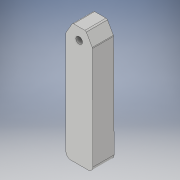
# Autodesk Inventor part: real arm
Saved by Autodesk Inventor 2019 (Build 230136000, 136)
## iProperties
Created: 2019-10-24
Part Number: real arm
Material: Generic
Document SubType Name: Modeling
Designer: robgr
Density: 1 g/cm^3
Appearance: Default
Author: robgr
Autodesk Inventor part; units mm, degrees
ref_plane "YZ Plane" through (0, 0, 0) normal (1, 0, 0) x (0, 1, 0)
ref_plane "XZ Plane" through (0, 0, 0) normal (0, 1, 0) x (-1, 0, 0)
ref_plane "XY Plane" through (0, 0, 0) normal (0, 0, 1) x (1, 0, 0)
sketch "Sketch1" plane through (0, 0, 0) normal (0, 0, 1) x (1, 0, 0)
  circle A0 centre (0, 0) radius 2
  line L0 (-8, 0) -> (-8, -65)
  line L1 (-8, -65) -> (8.3, -65)
  line L2 (8.3, -65) -> (8, 0)
  line L3 (-8, 0) -> (-4, 6.9282)
  line L4 (-4, 6.9282) -> (4, 6.9282)
  line L5 (4, 6.9282) -> (8, 0)
  dimension "d0" = 4
  dimension "d2" = 65
  dimension "d3" = 16.3
  constraints: 12 end point, 2 coincident, 1 centre point, 1 horizontal, 1 vertical, 6 other
  measures "d0" diameter of A0
  measures "d2" distance of L0.start L0.end
  measures "d3" distance of L0.end L1.end
extrude "Extrusion1" add sketch "Sketch1" along normal blind 12.75
fillet "Fillet1" radius 1 4 edges at (-4, 6.9282, 6.375) (4, 6.9282, 6.375) (8, 0, 6.375) (-8, 0, 6.375)
fillet "Fillet2" radius 3 2 edges at (8.3, -65, 6.375) (-8, -65, 6.375)
body "Solid1"
